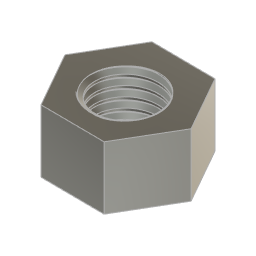
Hex nut (Autodesk Fusion 360 design; units mm, degrees)
Autodesk Fusion 360 part; units mm, degrees
note: some values were not read from the file. Chosen so that the rebuilt part matches the saved one: which face or edge a step refers to; where a thread starts.
sketch "Sketch1" plane through (0, 0, 0) normal (0, 0, 1) x (1, 0, 0)
  line L0 (-33.5403, -11.0504) -> (-41.8973, -25.2749)
  line L1 (-41.8973, -25.2749) -> (-33.757, -39.6245)
  line L2 (-33.757, -39.6245) -> (-17.2597, -39.7496)
  line L3 (-17.2597, -39.7496) -> (-8.9027, -25.5251)
  line L4 (-8.9027, -25.5251) -> (-17.043, -11.1755)
  line L5 (-17.043, -11.1755) -> (-33.5403, -11.0504)
  point P0 (-25.4, -25.4)
  dimension "d1" = 14.2875
  measures "d1" distance of P0 L5
extrude "Extrude1" add sketch "Sketch1" along normal blind 16.2719
hole "Hole1" at (-25.4, -25.4, 16.2719) direction (0, 0, -1) diameter 16.4592 end through all
thread "Thread1" "ANSI Unified Screw Threads 0.75 3/4-10 UNC 3B" major diameter 19.05 minor diameter 16.4668 pitch 2.54 angle 60 modelled right hand crest width 0.6893 on face at (-24.5806, -33.5887, 5.424) crest through (-25.4, -33.6334, 17.5419)
equation "d1 = ( 4.5 / 8 ) * 1 in"
equation "d2 = ( 41 / 64 ) * 1 in"
